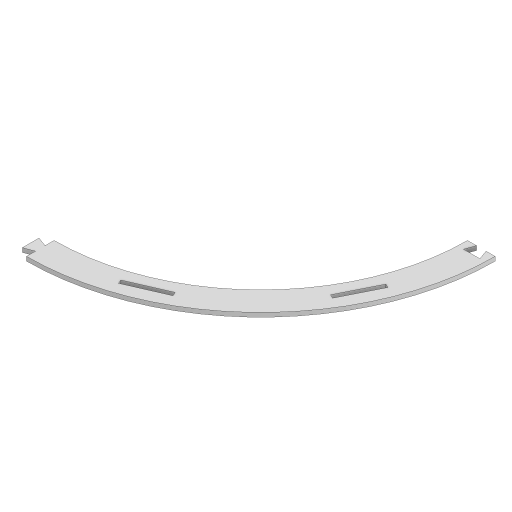
# Autodesk Inventor part: R30_CM_CIRCULO
Saved by Autodesk Inventor 2024.2 (Build 282272000, 272)
## iProperties
Created: 2024-10-01
Part Number: R30_CM_CIRCULO
Material: Generic
Document SubType Name: Modeling
Designer: jrcer
Density: 1 g/cm^3
Appearance: Default
Author: jrcer
Autodesk Inventor part; units mm, degrees
ref_plane "YZ Plane" through (0, 0, 0) normal (1, 0, 0) x (0, 1, 0)
ref_plane "XZ Plane" through (0, 0, 0) normal (0, 1, 0) x (-1, 0, 0)
ref_plane "XY Plane" through (0, 0, 0) normal (0, 0, 1) x (1, 0, 0)
sketch "Sketch1" plane through (0, 0, 0) normal (0, 1, 0) x (-1, 0, 0)
  circle A0 centre (0, 0) radius 150
  circle A1 centre (0, 0) radius 170
  line L0 (170, 0) -> (150, 0)
  line L1 (-170, 0) -> (-150, 0)
  line L2 (0, 0) -> (-150, 0) construction
  line L3 (0, 150) -> (0, 0) construction
  line L4 (0, 170) -> (0, 150)
  line L5 (-150, 0) -> (-170, 0)
  line L6 (-154, 7) -> (-166, 7)
  line L7 (-166, 7) -> (-163.4522, 0)
  line L8 (-154, 7) -> (-156.5478, 0)
  line L9 (-160, 0) -> (-160, 7) construction
  line L10 (-150.6597, 58.429) -> (-137.2628, 85.2715)
  line L11 (-137.2628, 85.2715) -> (-134.3996, 83.8425)
  line L12 (-134.3996, 83.8425) -> (-147.7965, 57)
  line L13 (-147.7965, 57) -> (-150.6597, 58.429)
  line L14 (-150.6597, 58.429) -> (-134.3996, 83.8425) construction
  line L15 (-137.2628, 85.2715) -> (-147.7965, 57) construction
  circle A2 centre (0, 0) radius 160 construction
  line L16 (-7, -154) -> (0, -156.5478)
  line L17 (-7, -166) -> (0, -163.4522)
  line L18 (-7, -154) -> (-7, -166)
  line L19 (154, -7) -> (156.5478, 0)
  line L20 (166, -7) -> (163.4522, 0)
  line L21 (154, -7) -> (166, -7)
  line L22 (7, 154) -> (0, 156.5478)
  line L23 (7, 166) -> (0, 163.4522)
  line L24 (7, 154) -> (7, 166)
  line L25 (-152.9695, -52.083) -> (-159.9609, -22.909)
  line L26 (-149.8576, -51.3372) -> (-152.9695, -52.083)
  line L27 (-156.849, -22.1633) -> (-149.8576, -51.3372)
  line L28 (-159.9609, -22.909) -> (-156.849, -22.1633)
  line L29 (-83.7031, -138.2248) -> (-107.8115, -120.3702)
  line L30 (-81.7986, -135.6532) -> (-83.7031, -138.2248)
  line L31 (-105.907, -117.7986) -> (-81.7986, -135.6532)
  line L32 (-107.8115, -120.3702) -> (-105.907, -117.7986)
  line L33 (24.7289, -159.6897) -> (-5.2159, -161.5088)
  line L34 (24.5348, -156.4956) -> (24.7289, -159.6897)
  line L35 (-5.41, -158.3147) -> (24.5348, -156.4956)
  line L36 (-5.2159, -161.5088) -> (-5.41, -158.3147)
  line L37 (121.5899, -106.434) -> (99.8202, -127.0757)
  line L38 (119.3882, -104.1119) -> (121.5899, -106.434)
  line L39 (97.6185, -124.7536) -> (119.3882, -104.1119)
  line L40 (99.8202, -127.0757) -> (97.6185, -124.7536)
  line L41 (161.5577, -3.3766) -> (158.1494, -33.1824)
  line L42 (158.3785, -3.0131) -> (161.5577, -3.3766)
  line L43 (154.9701, -32.8188) -> (158.3785, -3.0131)
  line L44 (158.1494, -33.1824) -> (154.9701, -32.8188)
  line L45 (125.9309, 101.2607) -> (142.4787, 76.2373)
  line L46 (123.2617, 99.4956) -> (125.9309, 101.2607)
  line L47 (139.8095, 74.4722) -> (123.2617, 99.4956)
  line L48 (142.4787, 76.2373) -> (139.8095, 74.4722)
  line L49 (31.3796, 158.517) -> (60.1406, 149.9847)
  line L50 (30.4694, 155.4491) -> (31.3796, 158.517)
  line L51 (59.2305, 146.9168) -> (30.4694, 155.4491)
  line L52 (60.1406, 149.9847) -> (59.2305, 146.9168)
  line L53 (-77.8546, 141.6014) -> (-50.3379, 153.5526)
  line L54 (-76.5798, 138.6663) -> (-77.8546, 141.6014)
  line L55 (-49.0631, 150.6175) -> (-76.5798, 138.6663)
  line L56 (-50.3379, 153.5526) -> (-49.0631, 150.6175)
  point P0 (160, 0)
  point P1 (-160, 0)
  point P2 (-142.5297, 71.1358)
  point P3 (-30.5894, 157.0487)
  point P4 (-149.2281, 57.7145)
  point P5 (-135.8312, 84.557)
  point P6 (-7, -160)
  point P7 (160, -7)
  point P8 (7, 160)
  point P9 (-151.4136, -51.7101)
  point P10 (-158.4049, -22.5361)
  point P11 (-82.7509, -136.939)
  point P12 (-106.8593, -119.0844)
  point P13 (24.6318, -158.0926)
  point P14 (-5.313, -159.9118)
  point P15 (120.4891, -105.2729)
  point P16 (98.7193, -125.9146)
  point P17 (159.9681, -3.1949)
  point P18 (156.5598, -33.0006)
  point P19 (124.5963, 100.3781)
  point P20 (141.1441, 75.3547)
  point P21 (30.9245, 156.983)
  point P22 (59.6856, 148.4508)
  point P23 (-77.2172, 140.1339)
  point P24 (-49.7005, 152.085)
  point P25 (-156.5478, 0)
  point P26 (0, 156.5478)
  point P27 (0, 163.4522)
  dimension "d0" = 300
  dimension "d1" = 340
  dimension "d4" = 90
  dimension "d5" = 7
  dimension "d6" = 70
  dimension "d8" = 12
  dimension "d13" = 3.2
  dimension "d14" = 30
  dimension "d15" = 50
  dimension "d20" = 320
  dimension "d23" = 360
  dimension "d27" = 360
  constraints: 114 end point, 11 point on circle, 8 midpoint, 3 centre point, 3 coincident, 3 parallel, 2 horizontal, 2 horizontal alignment, 2 perpendicular, 2 point on line, 2 vertical, 1 collinear, 1 equal length, 124 other
  measures "d0" diameter of A0
  measures "d1" diameter of A1
  measures "d4" angle of L2 L3
  measures "d5" distance between parallel lines of L6 L5
  measures "d6" angle of L7 L6
  measures "d8" distance of L6.start L6.end
  measures "d13" distance of L10.end L11.end
  measures "d14" distance of L11.end L12.end
  measures "d15" vertical distance of L12.end L6.start
  measures "d20" diameter of A2
extrude "Extrusion1" add sketch "Sketch1" along normal blind 3 contours A0 L1 L8 L6 L7 A1 L4 | L4 L23 L24 L22
body "Solid1"
